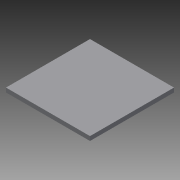
# Autodesk Inventor part: _BUILD PLATFORM
Saved by Autodesk Inventor 2013 (Build 170138000, 138)
## iProperties
Created: 2013-12-21
Part Number: _BUILD PLATFORM
Material: Generic
Document SubType Name: Modeling
Designer: employee
Density: 1 g/cm^3
Author: employee
Autodesk Inventor part; units mm, degrees
ref_plane "YZ Plane" through (0, 0, 0) normal (1, 0, 0) x (0, 1, 0)
ref_plane "XZ Plane" through (0, 0, 0) normal (0, 1, 0) x (-1, 0, 0)
ref_plane "XY Plane" through (0, 0, 0) normal (0, 0, 1) x (1, 0, 0)
sketch "Sketch1" plane through (0, 0, 0) normal (0, 0, 1) x (1, 0, 0)
  line L0 (-100, 100) -> (100, 100)
  line L1 (100, 100) -> (100, -100)
  line L2 (100, -100) -> (-100, -100)
  line L3 (-100, -100) -> (-100, 100)
  point P0 (0, 0)
  point P1 (-100, 0)
  point P2 (0, 100)
  dimension "d0" = 200
  constraints: 8 end point, 2 midpoint, 2 parallel, 2 perpendicular, 1 horizontal, 1 horizontal alignment, 1 vertical alignment
  measures "d0" distance of L0.start L0.end
extrude "Extrusion1" add sketch "Sketch1" along normal blind 10
body "Solid1"
